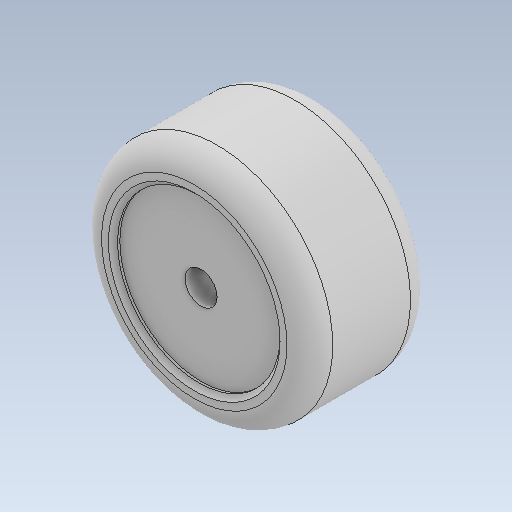
# Autodesk Inventor part: wheel_stand_in
Saved by Autodesk Inventor 2021.3 (Build 253353000, 353)
## iProperties
Created: 2021-10-12
Part Number: wheel_stand_in
Material: Generic
Document SubType Name: Modeling
Designer: nxf77172
Density: 1.93513 g/cm^3
Appearance: Default
Mass: 750 g
Surface Area: 329.746 cm^2
Volume: 387.57 cm^3
Author: nxf77172
Autodesk Inventor part; units mm, degrees
ref_plane "YZ Plane" through (0, 0, 0) normal (1, 0, 0) x (0, 1, 0)
ref_plane "XZ Plane" through (0, 0, 0) normal (0, 1, 0) x (-1, 0, 0)
ref_plane "XY Plane" through (0, 0, 0) normal (0, 0, 1) x (1, 0, 0)
sketch "Sketch2" plane through (0, 0, 0) normal (0, 0, 1) x (1, 0, 0)
  circle A0 centre (0, 0) radius 50.5
  circle A1 centre (0, 0) radius 47.5
  circle A2 centre (0, 0) radius 35.5
  circle A3 centre (0, 0) radius 7
  dimension "d0" = 101
  dimension "d1" = 3
  dimension "d2" = 15
  dimension "d3" = 14
  constraints: 4 centre point, 4 coincident
  measures "d0" diameter of A0
  measures "d1" radial gap between concentric circles of A0 A1
  measures "d2" radial gap between concentric circles of A0 A2
  measures "d3" diameter of A3
extrude "Extrusion1" add sketch "Sketch2" along normal blind 27 and the other way blind 27 contours A0 | A1 | A2
extrude "Extrusion2" cut sketch "Sketch2" against normal blind 3 from surface at 27 contours A2
extrude "Extrusion3" cut sketch "Sketch2" along normal blind 3 from surface at -27 contours A2
chamfer "Chamfer1" distance 2 angle 45 2 edges at (-35.5, 0, 27) (-35.5, 0, -27)
fillet "Fillet1" radius 10 2 edges at (-50.5, 0, -27) (-50.5, 0, 27)
body "Solid1"
